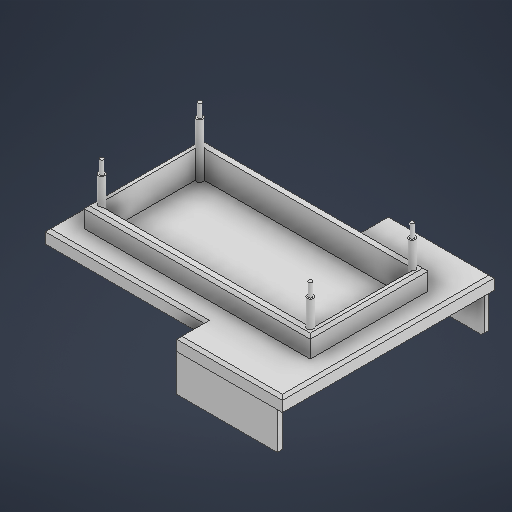
# Autodesk Inventor part: Buggy_Body_Wheel_Wells
Saved by Autodesk Inventor 2026.2 (Build 302298010, 298A)
## iProperties
Created: 2026-02-09
Part Number: Buggy_Body_Wheel_Wells
Material: Generic
Document SubType Name: Modeling
Designer: dm2166
Density: 1 g/cm^3
Appearance: Default
Mass: 237.324 g
Surface Area: 798.292 cm^2
Volume: 237.324 cm^3
Author: dm2166
Autodesk Inventor part; units mm, degrees
ref_plane "YZ Plane" through (0, 0, 0) normal (1, 0, 0) x (0, 1, 0)
ref_plane "XZ Plane" through (0, 0, 0) normal (0, 1, 0) x (-1, 0, 0)
ref_plane "XY Plane" through (0, 0, 0) normal (0, 0, 1) x (1, 0, 0)
sketch "Sketch1" plane through (0, 0, 0) normal (0, 1, 0) x (-1, 0, 0)
  line L0 (-85.5, -44.5) -> (85.5, -44.5)
  line L1 (85.5, -44.5) -> (85.5, 44.5)
  line L2 (85.5, 44.5) -> (-85.5, 44.5)
  line L3 (-85.5, 44.5) -> (-85.5, -44.5)
  line L4 (-85.5, -44.5) -> (85.5, 44.5) construction
  line L5 (85.5, -44.5) -> (-85.5, 44.5) construction
  line L6 (-81, -38.5) -> (81, -38.5)
  line L7 (81, -38.5) -> (81, 38.5)
  line L8 (81, 38.5) -> (-81, 38.5)
  line L9 (-81, 38.5) -> (-81, -38.5)
  line L10 (-81, -38.5) -> (81, 38.5) construction
  line L11 (81, -38.5) -> (-81, 38.5) construction
  line L12 (81, 38.5) -> (79.55, 38.5)
  line L13 (81, 37.05) -> (81, 38.5)
  circle A0 centre (79.55, 37.05) radius 1.45
  circle A1 centre (79.55, -37.05) radius 1.45
  circle A2 centre (-79.55, -38.5) radius 1.45
  circle A3 centre (-79.55, 38.472661) radius 1.45
  line L14 (81, -38.5) -> (81, -35.6)
  line L15 (-81, -38.5) -> (-78.1, -38.5)
  line L16 (-81, 38.5) -> (-81, 35.6)
  circle A4 centre (-79.55, 38.472661) radius 2.5
  line L17 (-95.556609, 0) -> (75.443391, 0)
  line L18 (0, 31.916696) -> (0, -57.083304)
  circle A5 centre (-79.55, -38.5) radius 2.5
  circle A6 centre (79.55, 37.05) radius 2.5
  circle A7 centre (79.55, -37.05) radius 2.5
  line L19 (140, 0) -> (-140, 0)
  line L20 (0, -112) -> (0, 112)
  line L21 (-100, 59.247527) -> (100, 59.247527)
  line L22 (100, 59.247527) -> (100, -59.247527)
  line L23 (100, -59.247527) -> (-100, -59.247527)
  line L24 (-100, -59.247527) -> (-100, 59.247527)
  line L25 (-100, 59.247527) -> (100, -59.247527) construction
  line L26 (100, 59.247527) -> (-100, -59.247527) construction
  line L27 (-100, 80) -> (-20, 80)
  line L28 (-20, 80) -> (-20, -80)
  line L29 (-20, -80) -> (-100, -80)
  line L30 (-100, -80) -> (-100, 80)
  line L31 (-100, 80) -> (-20, -80) construction
  line L32 (-20, 80) -> (-100, -80) construction
  line L33 (-79.55, 38.5) -> (-79.55, -38.5)
  point P0 (0, 0)
  point P1 (-80.999742, 38.5)
  point P2 (-81, 38.472661)
  point P3 (-81, -38.5)
  point P4 (-81, -38.5)
  point P5 (79.55, -38.5)
  point P6 (81, -37.05)
  point P7 (-60, 0)
  point P8 (-20, 59.247527)
  point P9 (-20, -59.247527)
  point P10 (-79.55, 0)
  point P11 (-78.100258, 38.5)
  dimension "d0" = 171
  dimension "d1" = 89
  dimension "d2" = 162
  dimension "d3" = 77
  dimension "d7" = 2.9
  dimension "d8" = 2.9
  dimension "d9" = 2.9
  dimension "d10" = 2.9
  dimension "d53" = 5
  dimension "d56" = 200
  dimension "d57" = 80
  dimension "d58" = 160
  dimension "d82" = 77
  constraints: 64 end point, 10 parallel, 9 midpoint, 8 centre point, 6 perpendicular, 5 horizontal, 4 point on line, 3 collinear, 3 concentric, 1 vertical
  measures "d0" distance of L2.end L1.end
  measures "d1" distance of L1.end L0.end
  measures "d2" distance of L8.end L7.end
  measures "d3" distance of L7.end L6.end
  measures "d7" diameter of A0
  measures "d8" diameter of A1
  measures "d9" diameter of A2
  measures "d10" diameter of A3
  measures "d53" diameter of A4
  measures "d56" distance of L22.end L23.end
  measures "d57" distance of L28.end L29.end
  measures "d58" distance of L27.end L28.end
  measures "d82" distance of L33.start L33.end
extrude "Extrusion1" add sketch "Sketch1" along normal blind 55 contours A2 L6 | L6 L33 A2 | L8 L33 A3 | A3 L8 | A2 L33 L6 | A1 | L33 L8 A3 | A0
extrude "Extrusion2" add sketch "Sketch1" along normal blind 4 contours L28 L17 L18 L6 | L6 A5 L33 L17 L28 | L17 L33 A5 L9 | L9 A4 L33 L17 | L18 L17 L19 L7 A7 L6 | L6 A2 L33 A5 | L28 L8 L20 L18 L17 | L17 L33 A4 L8 L28 | A5 L33 A2 L9 | A7 L7 A1 L6 | L18 L20 L8 A6 L7 L19 L17 | L6 L33 A2 | L8 L33 A3 | L9 A3 L33 A4 | A2 L33 L6 | L33 A3 L8 A4 | A1 L7 L6 | L33 L8 A3 | A6 L8 A0 L7 | A0 L8 L7
extrude "Extrusion3" add sketch "Sketch1" along normal blind 25 contours L3 L17 L9 A5 L6 L28 L0 | L28 L6 L18 L0 | L3 L2 L28 L8 A4 L9 L17 | L18 L6 A7 L7 L19 L1 L0 | A5 L9 A2 L6 | L2 L20 L8 L28 | L19 L7 A6 L8 L20 L2 L1 | L6 L7 A7 | A2 L6 | A4 L8 A3 L9 | A3 L8 | L7 L8 A6
chamfer "Chamfer1" distance 2 angle 45 4 edges at (0, 25, 44.5) (85.5, 25, 0) (0, 25, -44.5) (-85.5, 25, 0)
extrude "Extrusion11" add sketch "Sketch1" along normal blind 45 contours A5 L9 A2 L6 | L6 A2 L33 A5 | A5 L33 A2 L9 | A7 L7 A1 L6 | L6 L7 A7 | A2 L6 | L6 L33 A2 | L8 L33 A3 | A4 L8 A3 L9 | A3 L8 | L9 A3 L33 A4 | A2 L33 L6 | L33 A3 L8 A4 | A1 L7 L6 | A1 | L33 L8 A3 | A6 L8 A0 L7 | L7 L8 A6 | A0 L8 L7 | A0
extrude "Extrusion12" add sketch "Sketch1" along normal blind 10 contours L0 L28 L23 L24 L19 L17 L3 | L0 L18 L20 L23 L28 | L17 L19 L24 L21 L28 L2 L3 | L0 L1 L19 L22 L23 L20 L18 | L28 L29 L30 L23 | L28 L21 L20 L2 | L1 L2 L20 L21 L22 L19 | L21 L30 L27 L28
chamfer "Chamfer2" distance 2 angle 45 8 edges at (100, 10, 0) (60, 10, 80) (20, 10, 69.6238) (60, 10, -80) (20, 10, -69.6238) (-40, 10, -59.2475) (-40, 10, 59.2475) (-100, 10, 0)
sketch "Sketch4" plane through (0, 0, 0) normal (0, -1, 0) x (1, 0, 0)
  circle A0 centre (-11.267464, 0) radius 2
  circle A1 centre (-71.267465, 0) radius 2
  circle A2 centre (-41.267464, 30) radius 2
  circle A3 centre (-11.267464, 0) radius 1.9
  circle A4 centre (-71.267465, 0) radius 1.9
  circle A5 centre (-41.267464, 30) radius 1.9
  point P0 (0, 0)
  dimension "d64" = 3.8
  constraints: 3 centre point, 3 coincident, 2 equal radius
  measures "d64" diameter of A5
extrude "Extrusion13" add sketch "Sketch4" along normal blind 10 contours A3 | A4 | A5
sketch "Sketch6" plane through (0, 0, 0) normal (0, -1, 0) x (1, 0, 0)
  line L0 (96.084349, -75.000742) -> (96.084349, 74.999258)
  line L1 (96.084349, -76.250742) -> (23.584349, -76.250742)
  line L2 (23.584349, -76.250742) -> (23.584349, 76.249258)
  line L3 (23.584349, 76.249258) -> (96.084349, 76.249258)
  line L4 (96.084349, 76.249258) -> (96.084349, -76.250742)
  line L5 (96.084349, -76.250742) -> (23.584349, 76.249258) construction
  line L6 (23.584349, -76.250742) -> (96.084349, 76.249258) construction
  line L7 (20.000247, 79.999258) -> (100.000247, 79.999258)
  line L8 (20.000247, 59.246785) -> (20.000247, 79.999258)
  line L9 (20.000247, -80.000742) -> (20.000247, -59.248269)
  line L10 (100.000247, -80.000742) -> (20.000247, -80.000742)
  line L11 (96.084349, 76.249258) -> (96.084349, 79.999258)
  line L12 (96.084349, 79.999258) -> (20.000247, 79.999258)
  line L13 (20.000247, 79.999258) -> (20.000247, -80.000742)
  line L14 (20.000247, -80.000742) -> (96.084349, -80.000742)
  line L15 (96.084349, -80.000742) -> (96.084349, -76.250742)
  line L16 (20, 80) -> (100, 80)
  line L17 (100, -80) -> (20, -80)
  line L18 (20, -80) -> (20, -59.247527)
  point P0 (0, 0)
  point P1 (59.834349, -0.000742)
  point P2 (20.000247, -80)
  point P3 (96.084349, -80)
  dimension "d69" = 72.5
  dimension "d70" = 152.5
  constraints: 32 end point, 3 perpendicular, 3 point on line, 2 collinear, 2 midpoint, 2 parallel, 1 horizontal, 1 vertical
  measures "d69" distance of L2.end L3.end
  measures "d70" distance of L1.end L2.end
extrude "Extrusion14" add sketch "Sketch6" along normal blind 30 contours L15 L10 L9 L13 L8 L7 L11 L3 L2 L1
chamfer "Chamfer3" distance 2 angle 45 5 edges at (58.0423, -30, 79.9993) (20.0002, -30, -0.0004) (58.0423, -30, -80) (96.0843, -30, -78.1254) (96.0843, -30, 78.1243)
fillet "Fillet13" radius 2 4 edges at (20, 0, 69.6238) (20.0002, 0, -0.0004) (20.0001, 0, -80) (20, 0, -69.6238)
body "Solid1"
